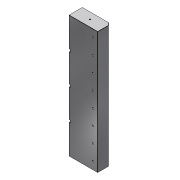
# Autodesk Inventor part: BC-10006
Saved by Autodesk Inventor 2016 (Build 200138000, 138)
## iProperties
Created: 2015-11-25
Part Number: BC-10006
Project: DIPOLO BC-3T- SIRIUS
Cost Center: 1504002005
Material: Aço Carbono AISI 1006
Document SubType Name: Modeling
Designer: Reinaldo.Basílio
Mass: 151025 g
Surface Area: 6523.2 cm^2
Volume: 19189.9 cm^3
Density: 7.87 g/cm^3
Appearance: Silver
Description: Compensador fixo do campo magnético.
RuleStatus: InUse
AfterMaterialChange0: file://_iMaterial
AfterAnyiPropertyChange0: file://_iMaterial
AfterDocNew0: file://_Naming_par
AfterDocNew1: file://_NameStart
AfterDocNew2: file://_NameStart1
AfterDocNew3: file://_Materiais
DocNumber: XXXXX-XXX-XXXX-00-001.ipt
Folder: .
Title: DIPOLO BC-3T- SIRIUS
Author: reinaldo.basilio
Subject: BC-10006
Autodesk Inventor part; units mm, degrees
ref_plane "YZ Plane" through (0, 0, 0) normal (1, 0, 0) x (0, 1, 0)
ref_plane "XZ Plane" through (0, 0, 0) normal (0, 1, 0) x (-1, 0, 0)
ref_plane "XY Plane" through (0, 0, 0) normal (0, 0, 1) x (1, 0, 0)
sketch "Sketch5" plane through (0, 0, 0) normal (0, 1, 0) x (-1, 0, 0)
  line L0 (50, 456.5) -> (-50, 456.5)
  line L1 (-50, 456.5) -> (-50, -456.5)
  line L2 (-50, -456.5) -> (50, -456.5)
  line L3 (50, -456.5) -> (50, 456.5)
  point P0 (0, 0)
  point P1 (50, 0)
  point P2 (0, 456.5)
  dimension "d8" = 100
  dimension "d9" = 913
  constraints: 8 end point, 2 midpoint, 2 parallel, 1 horizontal, 1 horizontal alignment, 1 perpendicular, 1 vertical alignment
  measures "d8" distance of L0.start L0.end
  measures "d9" distance of L0.end L1.end
extrude "Extrusion5" add sketch "Sketch5" along normal blind 215
sketch "Sketch7" plane through (-50, 0, -456.5) normal (-1, 0, 0) x (0, 0, 1)
  line L0 (0, 215) -> (913, 215) projected
  circle A0 centre (855.5, 180.25) radius 5.8396
  circle A1 centre (741.5, 180.25) radius 5.8396
  circle A2 centre (627.5, 180.25) radius 5.8396
  circle A3 centre (513.5, 180.25) radius 5.8396
  line L1 (456.5, 215) -> (456.5, 169.0746) construction
  circle A4 centre (57.5, 180.25) radius 5.8396
  circle A5 centre (171.5, 180.25) radius 5.8396
  circle A6 centre (285.5, 180.25) radius 5.8396
  circle A7 centre (399.5, 180.25) radius 5.8396
  line L2 (913, 0) -> (913, 215) projected
  point P0 (456.5, 0)
  point P1 (456.5, 0)
  dimension "d21" = 114
  dimension "d22" = 114
  dimension "d23" = 114
  dimension "d24" = 57
  dimension "d25" = 34.75
  dimension "d37" = 57.5
  constraints: 8 centre point, 4 symmetric about line, 3 equal radius, 3 horizontal alignment, 2 end point, 1 midpoint, 1 vertical, 4 other
  measures "d21" distance of A2.centre A3.centre
  measures "d22" distance of A2.centre A1.centre
  measures "d23" distance of A0.centre A1.centre
  measures "d24" distance from line of L1 A3.centre
  measures "d25" distance from line of L0 A0.centre
  measures "d37" distance from line of A0.centre L2
hole "Hole1" at (-50, 180.25, 399) at (-50, 180.25, 285) at (-50, 180.25, 171) at (-50, 180.25, 57) at (-50, 180.25, -57) at (-50, 180.25, -171) at (-50, 180.25, -285) at (-50, 180.25, -399) direction (1, 0, 0) diameter 12.5 end through all counterbore diameter 20 counterbore depth 60 clearance for "Socket Head Cap Screw DIN EN ISO 4762" size "M12" standard "DIN"
chamfer "Chamfer3" distance 20 angle 45 1 edges at (-50, 215, 0)
sketch "Sketch9" plane through (-50, 0, 456.5) normal (0, 0, 1) x (1, 0, 0)
  line L0 (0, 0) -> (100, 0) projected
  line L1 (100, 0) -> (100, 215) projected
  circle A0 centre (50, 107.5) radius 6
  point P0 (50, 0)
  point P1 (50, 0)
  point P2 (100, 107.5)
  dimension "d38" = 12
  constraints: 2 midpoint, 1 centre point, 1 horizontal alignment, 1 vertical alignment
  measures "d38" diameter of A0
hole "Hole2" at (0, 107.5, 456.5) direction (0, 0, -1) diameter 10.106 depth 30 tip angle 118 thread size "M12x1.75" class "6H" standard "ANSI Metric M Profile"
sketch "Sketch10" plane through (50, 0, -456.5) normal (0, 0, -1) x (-1, 0, 0)
  line L0 (0, 0) -> (0, 215) projected
  line L1 (0, 0) -> (100, 0) projected
  circle A0 centre (50, 107.5) radius 6
  point P0 (50, 0)
  point P1 (0, 107.5)
  point P2 (50, 0)
  dimension "d46" = 12
  constraints: 2 midpoint, 1 centre point, 1 horizontal alignment, 1 vertical alignment
  measures "d46" diameter of A0
hole "Hole3" at (0, 107.5, -456.5) direction (0, 0, 1) diameter 10.106 depth 30 tip angle 118 thread size "M12x1.75" class "6H" standard "ANSI Metric M Profile"
chamfer "Chamfer4" distance 1 angle 45 13 edges at (50, 215, 0) (10, 215, -456.5) (50, 107.5, -456.5) (-50, 97.5, -456.5) (0, 0, -456.5) (10, 215, 456.5) (-40, 205, 456.5) (-50, 97.5, 456.5) (50, 107.5, 456.5) (0, 0, 456.5) (50, 0, 0) (-50, 0, 0) (-40, 205, -456.5)
sketch "Sketch11" plane through (-50, 1, 455.5) normal (-1, 0, 0) x (0, 0, 1)
  line L0 (-217.5, -1) -> (-237.5, -1)
  line L1 (-237.5, -1) -> (-237.5, 9)
  line L2 (-237.5, 9) -> (-217.5, 9)
  line L3 (-217.5, 9) -> (-217.5, -1)
  line L4 (-445.5, -1) -> (-465.5, -1)
  line L5 (-465.5, -1) -> (-465.5, 9)
  line L6 (-465.5, 9) -> (-445.5, 9)
  line L7 (-445.5, 9) -> (-445.5, -1)
  line L8 (-911, -1) -> (0, -1) projected
  line L9 (-227.5, 9) -> (-227.5, 5.4206) construction
  line L10 (-455.5, -1) -> (-455.5, -35.8599) construction
  line L11 (-693.5, -1) -> (-673.5, -1)
  line L12 (-673.5, -1) -> (-673.5, 9)
  line L13 (-673.5, 9) -> (-693.5, 9)
  line L14 (-693.5, 9) -> (-693.5, -1)
  line L15 (-683.5, 9) -> (-683.5, 5.4206) construction
  point P0 (-455.5, 9)
  dimension "d57" = 20
  dimension "d58" = 10
  dimension "d59" = 10
  dimension "d60" = 20
  dimension "d61" = 228
  constraints: 30 end point, 6 symmetric about line, 4 parallel, 2 collinear, 2 horizontal, 2 midpoint, 2 perpendicular, 2 vertical, 1 point on line, 1 vertical alignment
  measures "d57" distance of L4.start L4.end
  measures "d58" distance of L4.end L5.end
  measures "d59" distance between parallel lines of L2 L8
  measures "d60" distance of L1.end L2.end
  measures "d61" distance of point (-455.5, 9) L9.start
extrude "Extrusion7" cut sketch "Sketch11" against normal through all
equation "\"d22\" = d21"
equation "\"d23\" = d21"
equation "\"d24\" = 0.5 * d21"
equation "\"d60\" = d57"
body "Solid5"
